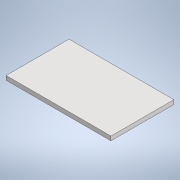
# Autodesk Inventor part: Part14
Saved by Autodesk Inventor 2022.3 (Build 263350000, 350)
## iProperties
Created: 2022-11-17
Part Number: Part14
Material: Generic
Document SubType Name: Modeling
Designer: komputer
Density: 1 g/cm^3
Appearance: Default
Author: komputer
Autodesk Inventor part; units mm, degrees
ref_plane "YZ Plane" through (0, 0, 0) normal (1, 0, 0) x (0, 1, 0)
ref_plane "XZ Plane" through (0, 0, 0) normal (0, 1, 0) x (-1, 0, 0)
ref_plane "XY Plane" through (0, 0, 0) normal (0, 0, 1) x (1, 0, 0)
sketch "Sketch1" plane through (0, 0, 0) normal (0, 0, 1) x (1, 0, 0)
  line L0 (-28.3248, 29.8117) -> (-13.1338, 22.5867)
  arc A0 (-13.1338, 22.5867) -> (-7.5529, 27.2374) centre (-11.4158, 26.1989) ccw
  arc A1 (7.5529, 27.2374) -> (13.1338, 22.5867) centre (11.4158, 26.1989) ccw
  line L1 (13.1338, 22.5867) -> (28.3248, 29.8117)
  circle A2 centre (-11.4158, 26.1989) radius 1.6
  circle A3 centre (20.9961, 37.6953) radius 1.6
  circle A4 centre (-20.9961, 37.6953) radius 1.6
  circle A5 centre (11.4158, 26.1989) radius 1.6
  line L2 (50, 45.5218) -> (11.4158, 45.5218)
  line L3 (11.4158, 45.5218) -> (11.4158, 48.5218)
  line L4 (11.4158, 48.5218) -> (-11.4158, 48.5218)
  line L5 (-11.4158, 48.5218) -> (-11.4158, 45.5218)
  line L6 (-11.4158, 45.5218) -> (-50, 45.5218)
  line L7 (-50, 45.5218) -> (-50, -40)
  line L8 (-50, -40) -> (50, -40)
  line L9 (50, 45.5218) -> (50, -40)
  line L10 (-50, 21.0398) -> (50, 21.0398)
  line L11 (-50, 21.0398) -> (50, 21.0398)
  line L12 (50, 21.0398) -> (50, 17.0398)
  line L13 (50, 17.0398) -> (-50, 17.0398)
  line L14 (-50, 17.0398) -> (-50, 21.0398)
  ellipse E0 centre (-80.335, 109.4905) end of major axis (-69.5799, 118.453) minor radius 2.0831
  ellipse E1 centre (80.9138, 109.0081) end of major axis (91.6689, 100.0455) minor radius 2.0831
  point P0 (0, 0)
  point P1 (-50, 17.0398)
extrude "Extrusion1" add sketch "Sketch1" along normal blind 60 contours L9 L13 L7 L10
sketch "Sketch2" plane through (-50, 21.0398, 0) normal (0, 1, 0) x (1, 0, 0)
  line L0 (100, 0) -> (0, 0) projected
  line L1 (0, 0) -> (0, -60) projected
  line L2 (100, -60) -> (0, -60) projected
  line L3 (100, 0) -> (100, -60) projected
  ellipse E0 centre (103.0593, -17.711) end of major axis (100.5424, -28.4192) minor radius 8.3564 projected
  line L4 (74.521, -31.0293) -> (129.597, -43.9743) projected
  line L5 (74.521, -31.0293) -> (75.4379, -21.5102) projected
  line L6 (25.4921, -31.1653) -> (-29.5839, -44.1102) projected
  line L7 (22.9377, -28.1696) -> (-27.3904, -39.9986) projected
  line L8 (24.5621, -21.5102) -> (25.4921, -31.1653) projected
  ellipse E1 centre (79.9812, -12.3391) end of major axis (77.0068, -24.9943) minor radius 9.8757 (81.4774, -24.7198) -> (76.0998, -24.7198) ccw projected
  ellipse E2 centre (20.0188, -12.3391) end of major axis (22.9932, -24.9943) minor radius 9.8757 (23.9002, -24.7198) -> (18.5226, -24.7198) ccw projected
  ellipse E3 centre (66.6015, -11) end of major axis (66.6015, -15) minor radius 2.5607 (64.0407, -11) -> (69.1622, -11) ccw projected
  ellipse E4 centre (33.3985, -11) end of major axis (33.3985, -7) minor radius 2.5607 (30.8378, -11) -> (35.9593, -11) ccw projected
  line L9 (42.4471, -5) -> (38.0799, -5) projected
  line L10 (64.0407, -5) -> (64.0407, -11) projected
  line L11 (35.9593, -5) -> (35.9593, -11) projected
  point P0 (50, 0)
  point P1 (61.9201, -5)
  constraints: 6 other
body "Solid1"
